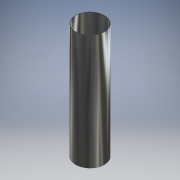
# Autodesk Inventor part: Tubo
Saved by Autodesk Inventor 2016 (Build 200138000, 138)
## iProperties
Created: 2017-04-03
Part Number: Tubo
Material: Nickel-Copper Alloy 400
Document SubType Name: Modeling
Designer: Marcelo
Mass: 4635.9 g
Surface Area: 10013.4 cm^2
Volume: 525.017 cm^3
Density: 8.83 g/cm^3
Appearance: Chrome - Polished
Author: Marcelo
Autodesk Inventor part; units mm, degrees
ref_plane "YZ Plane" through (0, 0, 0) normal (1, 0, 0) x (0, 1, 0)
ref_plane "XZ Plane" through (0, 0, 0) normal (0, 1, 0) x (-1, 0, 0)
ref_plane "XY Plane" through (0, 0, 0) normal (0, 0, 1) x (1, 0, 0)
sketch "Sketch1" plane through (0, 0, 0) normal (0, 0, 1) x (1, 0, 0)
  circle A0 centre (0, 0) radius 100
  circle A1 centre (0, 0) radius 98.95
  dimension "d0" = 200
  dimension "d1" = 197.9
  constraints: 2 centre point, 2 coincident
  measures "d0" diameter of A0
  measures "d1" diameter of A1
extrude "Extrusion1" add sketch "Sketch1" along normal blind 800
body "Solid1"
